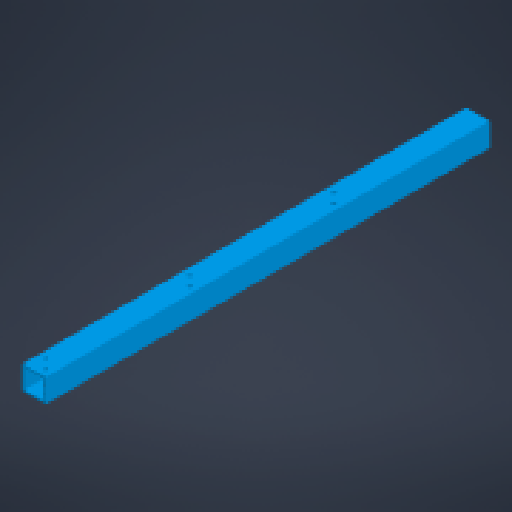
# Autodesk Inventor part: square_box_section
Saved by Autodesk Inventor 2024 (Build 280153000, 153)
## iProperties
Created: 2023-04-13
Part Number: square_box_section
Material: Типовые
Document SubType Name: Modeling
Designer: user
Density: 1 g/cm^3
Appearance: По умолчанию
Author: user
Autodesk Inventor part; units mm, degrees
ref_plane "YZ Plane" through (0, 0, 0) normal (1, 0, 0) x (0, 1, 0)
ref_plane "XZ Plane" through (0, 0, 0) normal (0, 1, 0) x (-1, 0, 0)
ref_plane "XY Plane" through (0, 0, 0) normal (0, 0, 1) x (1, 0, 0)
sketch "Эскиз1" plane through (0, 0, 0) normal (0, 0, 1) x (1, 0, 0)
  line L0 (0, 0) -> (20, 0)
  line L1 (20, 0) -> (20, 20)
  line L2 (20, 20) -> (0, 20)
  line L3 (0, 20) -> (0, 0)
  line L4 (1.5, 1.5) -> (18.5, 1.5)
  line L5 (18.5, 1.5) -> (18.5, 18.5)
  line L6 (18.5, 18.5) -> (1.5, 18.5)
  line L7 (1.5, 18.5) -> (1.5, 1.5)
  point P0 (10, 18.5)
  point P1 (10, 20)
  point P2 (18.5, 10)
  point P3 (20, 10)
  dimension "d2" = 20
  dimension "d3" = 1.5
  constraints: 16 end point, 4 midpoint, 4 parallel, 4 perpendicular, 2 horizontal, 1 horizontal alignment, 1 vertical alignment
  measures "d2" distance of L1.end L2.end
  measures "d3" horizontal distance of L2.end L6.end
extrude "Выдавливание1" add sketch "Эскиз1" along normal blind 380
sketch "Эскиз6" plane through (0, 0, 0) normal (0, -1, 0) x (1, 0, 0)
  circle A0 centre (14, 374) radius 2
  circle A1 centre (6, 366) radius 2
  line L0 (20, 360) -> (0, 360) construction
  line L1 (14, 374) -> (14, 380) construction
  line L2 (14, 374) -> (20, 374) construction
  line L3 (6, 366) -> (0, 366) construction
  line L4 (6, 366) -> (6, 360) construction
  line L5 (1.5, 0) -> (18.5, 0) construction
  line L6 (0, 380) -> (20, 380) construction
  line L7 (0, 0) -> (0, 380) construction
  line L8 (0, 257) -> (20, 257) construction
  line L9 (20, 0) -> (20, 380) construction
  line L10 (0, 0) -> (0, 380) construction
  line L11 (0, 237) -> (20, 237) construction
  circle A2 centre (6, 243) radius 2
  circle A3 centre (14, 251) radius 2
  line L12 (6, 243) -> (6, 237) construction
  line L13 (14, 251) -> (14, 257) construction
  line L14 (0, 134) -> (20, 134) construction
  line L15 (0, 114) -> (20, 114) construction
  circle A4 centre (6, 120) radius 2
  circle A5 centre (14, 128) radius 2
  line L16 (6, 120) -> (6, 114) construction
  line L17 (14, 128) -> (14, 134) construction
  dimension "d13" = 20
  dimension "d14" = 6
  dimension "d20" = 4
  dimension "d21" = 123
  dimension "d22" = 20
  dimension "d23" = 20
  dimension "d25" = 123
  constraints: 26 end point, 18 point on line, 9 perpendicular, 7 equal length, 6 centre point, 5 equal radius, 4 vertical alignment, 3 horizontal, 1 vertical
  measures "d13" distance of L0.start L6.end
  measures "d14" distance of L3.start L3.end
  measures "d20" diameter of A1
  measures "d21" distance of L6.end L8.end
  measures "d22" distance of L11.start L8.start
  measures "d23" distance of L15.start L14.start
  measures "d25" distance of L8.start L14.start
extrude "Выдавливание3" cut sketch "Эскиз6" against normal through all
